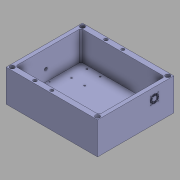
# Autodesk Inventor part: podstawa_2
Saved by Autodesk Inventor 2021 (Build 250183000, 183)
## iProperties
Created: 2022-06-23
Part Number: podstawa_2
Material: PC/ABS Plastic
Document SubType Name: Modeling
Designer: agnpi
Density: 0.357273 g/cm^3
Appearance: Olive Green
Author: agnpi
Autodesk Inventor part; units mm, degrees
ref_plane "YZ Plane" through (0, 0, 0) normal (1, 0, 0) x (0, 1, 0)
ref_plane "XZ Plane" through (0, 0, 0) normal (0, 1, 0) x (-1, 0, 0)
ref_plane "XY Plane" through (0, 0, 0) normal (0, 0, 1) x (1, 0, 0)
sketch "Sketch1" plane through (0, 0, 0) normal (0, 1, 0) x (-1, 0, 0)
  line L0 (179.2, 0) -> (-179.2, 0) projected
  line L1 (0, -144.2) -> (0, 144.2) projected
  line L2 (-120, 95) -> (120, 95)
  line L3 (120, 95) -> (120, -95)
  line L4 (120, -95) -> (-120, -95)
  line L5 (-120, -95) -> (-120, 95)
  line L6 (-120, 95) -> (120, -95) construction
  line L7 (120, 95) -> (-120, -95) construction
  line L8 (-128, 103) -> (128, 103)
  line L9 (128, 103) -> (128, -103)
  line L10 (128, -103) -> (-128, -103)
  line L11 (-128, -103) -> (-128, 103)
  point P0 (0, 0)
  dimension "d0" = 240
  dimension "d1" = 190
  dimension "d2" = 8
  dimension "d3" = 8
  dimension "d4" = 8
  dimension "d5" = 8
  constraints: 20 end point, 3 parallel, 3 perpendicular, 2 horizontal, 2 midpoint
  measures "d0" distance of L3.end L4.end
  measures "d1" distance of L2.end L3.end
  measures "d2" distance between parallel lines of L2 L8
  measures "d3" distance between parallel lines of L10 L4
  measures "d4" distance between parallel lines of L11 L5
  measures "d5" distance between parallel lines of L9 L3
extrude "Extrusion1" add sketch "Sketch1" along normal blind 8 contours L3 L4 L1 L0 | L0 L1 L2 L3 | L1 L4 L5 L0 | L0 L5 L2 L1
extrude "Extrusion2" add sketch "Sketch1" along normal blind 85 contours L9 L10 L1 L4 L3 L0 | L0 L3 L2 L1 L8 L9 | L1 L2 L5 L0 L11 L8 | L10 L11 L0 L5 L4 L1
move faces "Move1" translate (-16, 0, 0) faces at (120, 33.6667, -31.6667)
move faces "Move5" translate (-8, 0, 0) faces at (128, 28.3333, 34.3333)
move faces "Move6" translate (-8, 0, 0) faces at (120, 28.3333, 34.3333)
move faces "Move7" translate (0, 0, -8) faces at (-45.3333, 59.3333, 95)
move faces "Move8" translate (0, 0, -8) faces at (-48, 28.3333, 103)
move faces "Move9" translate (0, 0, -8) faces at (-45.3333, 59.3333, 87)
move faces "Move10" translate (0, 0, -8) faces at (-48, 28.3333, 95)
thicken "Thicken1" operation add thickness 3 both sides no extend neighbours yes toward (0, 0, 1) faces at (-48, 28.3333, 87)
thicken "Thicken3" operation add thickness 3 both sides no extend neighbours yes toward (0, 0, -1) faces at (32, 28.3333, -103)
sketch "Sketch5" plane through (0, 8, 0) normal (0, 1, 0) x (1, 0, 0)
  line L0 (-120, -79) -> (-120, 95) projected
  line L1 (-120, 95) -> (104, 95) projected
  line L2 (-120, 89.3431) -> (-114.3431, 95)
  line L3 (-120, 89.3431) -> (-120, 95)
  line L4 (98.3431, 95) -> (104, 89.3431)
  line L5 (104, 95) -> (104, -79) projected
  line L6 (-120, -73.3431) -> (-114.3431, -79)
  line L7 (104, -79) -> (-120, -79) projected
  line L8 (98.3431, -79) -> (104, -73.3431)
  point P0 (0, 0)
  dimension "d69" = 45
  dimension "d70" = 8
  dimension "d73" = 8
  dimension "d74" = 45
  dimension "d75" = 8
  dimension "d76" = 45
  dimension "d77" = 8
  dimension "d78" = 45
  constraints: 10 end point, 8 point on line, 1 collinear
  measures "d69" angle of L2 L0
  measures "d70" distance of L2.start L2.end
  measures "d73" distance of L4.start L4.end
  measures "d74" angle of L5 L4
  measures "d75" distance of L6.start L6.end
  measures "d76" angle of L7 L6
  measures "d77" distance of L8.start L8.end
  measures "d78" angle of L7 L8
thicken "Thicken4" operation add thickness 1 both sides no extend neighbours yes toward (1, 0, 0) faces at (-120, 59.3333, 21)
thicken "Thicken5" operation add thickness 1 both sides no extend neighbours yes toward (-1, 0, 0) faces at (104, 33.6667, 21)
extrude "Extrusion6" add sketch "Sketch5" along normal up to surface (77 mm away) contours L0 L6 L7 | L0 L1 L2 | L8 L5 L7 | L1 L5 L4
sketch "Sketch7" plane through (0, 8, 0) normal (0, 1, 0) x (1, 0, 0)
  line L0 (-119, -74.3431) -> (-119, 90.3431) projected
  line L1 (-114.3431, 95) -> (98.3431, 95) projected
  point P0 (0, 0)
  point P1 (-94.5, 86.37)
  point P2 (-59.5, 86.37)
  point P3 (-94.5, 45.37)
  point P4 (-59.5, 45.37)
  dimension "d95" = 24.5
  dimension "d96" = 24.5
  dimension "d97" = 41
  dimension "d98" = 35
  dimension "d99" = 35
  dimension "d100" = 8.63
  dimension "d101" = 8.63
  dimension "d102" = 41
  measures "d95" distance from line of L0 point (-94.5, 86.37)
  measures "d96" distance from line of L0 point (-94.5, 45.37)
  measures "d97" distance of point (-94.5, 86.37) point (-94.5, 45.37)
  measures "d98" distance of point (-59.5, 45.37) point (-94.5, 45.37)
  measures "d99" distance of point (-59.5, 86.37) point (-94.5, 86.37)
  measures "d100" distance from line of L1 point (-59.5, 86.37)
  measures "d101" distance from line of L1 point (-94.5, 86.37)
  measures "d102" distance of point (-59.5, 45.37) point (-59.5, 86.37)
hole "Hole2" at (-94.5, 8, -86.37) at (-59.5, 8, -86.37) at (-94.5, 8, -45.37) at (-59.5, 8, -45.37) direction (0, -1, 0) diameter 4 end through all
sketch "Sketch8" plane through (0, 8, 0) normal (0, 1, 0) x (1, 0, 0)
  line L0 (-114.3431, 95) -> (98.3431, 95) projected
  line L1 (103, 90.3431) -> (103, -74.3431) projected
  point P0 (0, 0)
  point P1 (29, 66.38)
  point P2 (71, 66.37)
  point P3 (38.2, 51.57)
  point P4 (66.91, 51.57)
  dimension "d110" = 28.71
  dimension "d111" = 28.63
  dimension "d112" = 28.62
  dimension "d113" = 43.43
  dimension "d114" = 43.43
  dimension "d115" = 74
  dimension "d116" = 42
  dimension "d117" = 64.8
  measures "d110" distance of point (66.91, 51.57) point (38.2, 51.57)
  measures "d111" distance from line of L0 point (71, 66.37)
  measures "d112" distance from line of L0 point (29, 66.38)
  measures "d113" distance from line of L0 point (66.91, 51.57)
  measures "d114" distance from line of L0 point (38.2, 51.57)
  measures "d115" distance from line of L1 point (29, 66.38)
  measures "d116" distance of point (71, 66.37) point (29, 66.38)
  measures "d117" distance from line of L1 point (38.2, 51.57)
hole "Hole3" at (29, 8, -66.38) at (71, 8, -66.37) at (38.2, 8, -51.57) at (66.91, 8, -51.57) direction (0, -1, 0) diameter 4 end through all
sketch "Sketch9" plane through (0, 8, 0) normal (0, 1, 0) x (1, 0, 0)
  line L0 (103, 90.3431) -> (103, -74.3431) projected
  line L1 (98.3431, -79) -> (-114.3431, -79) projected
  point P0 (0, 0)
  point P1 (35, 18.8)
  point P2 (70, 18.8)
  point P3 (35, -14.2)
  point P4 (70, -14.2)
  dimension "d125" = 33
  dimension "d126" = 33
  dimension "d127" = 35
  dimension "d128" = 35
  dimension "d129" = 33
  dimension "d130" = 33
  dimension "d131" = 64.8
  dimension "d132" = 64.8
  measures "d125" distance from line of L0 point (70, 18.8)
  measures "d126" distance from line of L0 point (70, -14.2)
  measures "d127" distance of point (70, 18.8) point (35, 18.8)
  measures "d128" distance of point (70, -14.2) point (35, -14.2)
  measures "d129" distance of point (35, -14.2) point (35, 18.8)
  measures "d130" distance of point (70, -14.2) point (70, 18.8)
  measures "d131" distance from line of L1 point (35, -14.2)
  measures "d132" distance from line of L1 point (70, -14.2)
hole "Hole4" at (35, 8, -18.8) at (70, 8, -18.8) at (35, 8, 14.2) at (70, 8, 14.2) direction (0, -1, 0) diameter 4 end through all
sketch "Sketch10" plane through (0, 8, 0) normal (0, 1, 0) x (1, 0, 0)
  line L0 (-119, -74.3431) -> (-119, 90.3431) projected
  line L1 (98.3431, -79) -> (-114.3431, -79) projected
  point P0 (0, 0)
  point P1 (-115, 7.85)
  point P2 (-115, -4.15)
  dimension "d140" = 4
  dimension "d141" = 4
  dimension "d142" = 74.85
  dimension "d143" = 12
  measures "d140" distance from line of L0 point (-115, -4.15)
  measures "d141" distance from line of L0 point (-115, 7.85)
  measures "d142" distance from line of L1 point (-115, -4.15)
  measures "d143" distance of point (-115, 7.85) point (-115, -4.15)
hole "Hole5" at (-115, 8, -7.85) at (-115, 8, 4.15) direction (0, -1, 0) diameter 3 end through all
move faces "Move21" translate (0, 0, 3) faces at (-48, 28.3333, 90)
move faces "Move22" translate (0, 0, -3) faces at (-48, 56.6667, -106)
move faces "Move23" translate (1, 0, 0) faces at (112, 56.6667, -41.6667)
move faces "Move24" translate (-1, 0, 0) faces at (-128, 28.3333, -41.6667)
sketch "Sketch15" plane through (0, 85, 0) normal (0, 1, 0) x (1, 0, 0)
  circle A0 centre (-121, 101) radius 6
  line L0 (113, 109) -> (-129, 109) projected
  line L1 (-129, 109) -> (-129, -93) projected
  circle A1 centre (105, 101) radius 6
  line L2 (113, -93) -> (113, 109) projected
  circle A2 centre (105, -85) radius 6
  line L3 (-129, -93) -> (113, -93) projected
  circle A3 centre (-121, -85) radius 6
  point P0 (0, 0)
  dimension "d204" = 12
  dimension "d205" = 8
  dimension "d206" = 8
  dimension "d207" = 12
  dimension "d208" = 8
  dimension "d209" = 8
  dimension "d210" = 12
  dimension "d211" = 8
  dimension "d212" = 8
  dimension "d213" = 12
  dimension "d214" = 8
  dimension "d215" = 8
  constraints: 4 centre point
  measures "d204" diameter of A0
  measures "d205" distance from line of L0 A0.centre
  measures "d206" distance from line of L1 A0.centre
  measures "d207" diameter of A1
  measures "d208" distance from line of L2 A1.centre
  measures "d209" distance from line of L0 A1.centre
  measures "d210" diameter of A2
  measures "d211" distance from line of L2 A2.centre
  measures "d212" distance from line of L3 A2.centre
  measures "d213" diameter of A3
  measures "d214" distance from line of L3 A3.centre
  measures "d215" distance from line of L1 A3.centre
extrude "Extrusion7" cut sketch "Sketch15" against normal blind 15 contours A0 | A1 | A2 | A3
sketch "Sketch16" plane through (-129, 0, -109) normal (-1, 0, 0) x (0, 0, 1)
  circle A0 centre (107.1, 38) radius 4
  line L0 (202, 0) -> (202, 85) projected
  line L1 (0, 0) -> (202, 0) projected
  point P0 (109, 0)
  dimension "d218" = 8
  dimension "d219" = 94.9
  dimension "d220" = 38
  constraints: 1 centre point
  measures "d218" diameter of A0
  measures "d219" distance from line of L0 A0.centre
  measures "d220" distance from line of L1 A0.centre
extrude "Extrusion8" cut sketch "Sketch16" against normal up to surface (10 mm away)
sketch "Sketch17" plane through (0, 85, 0) normal (0, 1, 0) x (1, 0, 0)
  circle A0 centre (-60, -86) radius 4.5
  circle A1 centre (105, -85) radius 6 projected
  line L0 (-129, -93) -> (113, -93) projected
  circle A2 centre (-60, 102) radius 4.5
  line L1 (113, 109) -> (-129, 109) projected
  circle A3 centre (105, 101) radius 6 projected
  circle A4 centre (-121, -85) radius 6 projected
  circle A5 centre (-121, 101) radius 6 projected
  point P0 (0, 0)
  dimension "d223" = 9
  dimension "d225" = 7
  dimension "d226" = 9
  dimension "d227" = 7
  dimension "d231" = 61
  dimension "d232" = 61
  constraints: 2 centre point
  measures "d223" diameter of A0
  measures "d225" distance from line of L0 A0.centre
  measures "d226" diameter of A2
  measures "d227" distance from line of L1 A2.centre
  measures "d231" horizontal distance of A4.centre A0.centre
  measures "d232" horizontal distance of A5.centre A2.centre
extrude "Extrusion9" cut sketch "Sketch17" against normal blind 15 contours A0 | A2
sketch "Sketch18" plane through (0, 85, 0) normal (0, 1, 0) x (1, 0, 0)
  circle A0 centre (-15, -86) radius 4
  circle A1 centre (-15, 102) radius 4
  circle A2 centre (105, -85) radius 6 projected
  circle A3 centre (105, 101) radius 6 projected
  line L0 (113, 109) -> (-129, 109) projected
  line L1 (-129, -93) -> (113, -93) projected
  point P0 (0, 0)
  dimension "d233" = 8
  dimension "d234" = 8
  dimension "d235" = 120
  dimension "d236" = 120
  dimension "d237" = 7
  dimension "d238" = 7
  constraints: 2 centre point
  measures "d233" diameter of A0
  measures "d234" diameter of A1
  measures "d235" horizontal distance of A0.centre A2.centre
  measures "d236" horizontal distance of A1.centre A3.centre
  measures "d237" distance from line of L0 A1.centre
  measures "d238" distance from line of L1 A0.centre
extrude "Extrusion10" cut sketch "Sketch18" against normal blind 15 contours A0 | A1
sketch "Sketch19" plane through (-129, 0, -109) normal (-1, 0, 0) x (0, 0, 1)
  line L0 (162, 45) -> (182, 45)
  line L1 (182, 45) -> (182, 25)
  line L2 (182, 25) -> (162, 25)
  line L3 (162, 25) -> (162, 45)
  line L4 (202, 0) -> (202, 85) projected
  line L5 (0, 0) -> (202, 0) projected
  point P0 (109, 0)
  dimension "d241" = 20
  dimension "d242" = 20
  dimension "d243" = 45
  dimension "d244" = 25
  constraints: 8 end point, 2 parallel, 1 horizontal, 1 perpendicular
  measures "d241" distance between parallel lines of L4 L1
  measures "d242" distance between parallel lines of L3 L1
  measures "d243" distance between parallel lines of L5 L0
  measures "d244" distance between parallel lines of L5 L2
extrude "Extrusion11" cut sketch "Sketch19" against normal up to surface (10 mm away)
sketch "Sketch20" plane through (103, 8, -90.3431) normal (-1, 0, 0) x (0, 0, 1)
  line L0 (20, 66) -> (45.5, 66)
  line L1 (45.5, 66) -> (45.5, 63)
  line L2 (45.5, 63) -> (20, 63)
  line L3 (20, 63) -> (20, 66)
  line L4 (20, 63) -> (17, 63)
  line L5 (17, 63) -> (17, 37.5)
  line L6 (17, 37.5) -> (20, 37.5)
  line L7 (20, 37.5) -> (20, 63)
  line L8 (20, 37.5) -> (45.5, 37.5)
  line L9 (45.5, 37.5) -> (45.5, 34.5)
  line L10 (45.5, 34.5) -> (20, 34.5)
  line L11 (20, 34.5) -> (20, 37.5)
  line L12 (45.5, 63) -> (48.5, 63)
  line L13 (48.5, 63) -> (48.5, 37.5)
  line L14 (48.5, 37.5) -> (45.5, 37.5)
  line L15 (45.5, 37.5) -> (45.5, 63)
  line L16 (0, 77) -> (164.6863, 77) projected
  line L17 (0, 77) -> (0, 0) projected
  point P0 (90.3431, -8)
  dimension "d247" = 3
  dimension "d248" = 14
  dimension "d249" = 25.5
  dimension "d250" = 25.5
  dimension "d251" = 25.5
  dimension "d252" = 25.5
  dimension "d253" = 3
  dimension "d254" = 3
  dimension "d255" = 3
  dimension "d256" = 20
  constraints: 32 end point, 8 parallel, 4 horizontal, 4 perpendicular, 1 point on line
  measures "d247" distance between parallel lines of L2 L0
  measures "d248" distance between parallel lines of L16 L2
  measures "d249" distance of L1.end L2.end
  measures "d250" distance of L4.end L5.end
  measures "d251" distance of L9.end L10.end
  measures "d252" distance of L12.end L13.end
  measures "d253" distance between parallel lines of L8 L10
  measures "d254" distance between parallel lines of L7 L5
  measures "d255" distance between parallel lines of L13 L15
  measures "d256" distance from line of L17 L2.end
extrude "Extrusion12" add sketch "Sketch20" along normal blind 3 contours L0 L1 L2 L3 | L7 L6 L5 L4 | L12 L13 L14 L15 | L8 L9 L10 L11
sketch "Sketch21" plane through (103, 45.5, -70.3431) normal (-1, 0, 0) x (0, 0, 1)
  circle A0 centre (2.75, 2.75) radius 1.5
  circle A1 centre (2.75, 22.75) radius 1.5
  circle A2 centre (22.75, 22.75) radius 1.5
  circle A3 centre (22.75, 2.75) radius 1.5
  line L0 (0, 25.5) -> (25.5, 25.5) projected
  line L1 (0, 0) -> (0, 25.5) projected
  line L2 (0, 0) -> (25.5, 0) projected
  line L3 (25.5, 25.5) -> (25.5, 0) projected
  point P0 (70.3431, -45.5)
  dimension "d259" = 3
  dimension "d260" = 3
  dimension "d261" = 3
  dimension "d262" = 3
  dimension "d263" = 2.75
  dimension "d264" = 2.75
  dimension "d265" = 2.75
  dimension "d266" = 2.75
  dimension "d267" = 2.75
  dimension "d268" = 2.75
  dimension "d269" = 2.75
  dimension "d270" = 2.75
  constraints: 4 centre point
  measures "d259" diameter of A0
  measures "d260" diameter of A1
  measures "d261" diameter of A2
  measures "d262" diameter of A3
  measures "d263" distance from line of L0 A1.centre
  measures "d264" distance from line of L1 A1.centre
  measures "d265" distance from line of L2 A0.centre
  measures "d266" distance from line of L1 A0.centre
  measures "d267" distance from line of L0 A2.centre
  measures "d268" distance from line of L3 A3.centre
  measures "d269" distance from line of L2 A3.centre
  measures "d270" distance from line of L3 A2.centre
extrude "Extrusion13" cut sketch "Sketch21" against normal through all contours A0 | A1 | A2 | A3
sketch "Sketch22" plane through (113, 0, 93) normal (1, 0, 0) x (0, 0, -1)
  line L0 (137.8431, 71) -> (137.8431, 74) projected
  line L1 (163.3431, 71) -> (163.3431, 45.5) projected
  line L2 (137.8431, 71) -> (163.3431, 71)
  line L3 (163.3431, 71) -> (163.3431, 45.5)
  line L4 (163.3431, 45.5) -> (137.8431, 45.5)
  line L5 (137.8431, 45.5) -> (137.8431, 71)
  circle A0 centre (150.5931, 58.25) radius 6
  circle A1 centre (150.5931, 58.25) radius 11.5
  line L6 (146.0144, 62.1275) -> (142.0931, 65.996)
  line L7 (147.1208, 63.1431) -> (143.174, 67.0367)
  line L8 (144.9458, 56.2234) -> (139.6349, 54.7618)
  line L9 (144.6194, 57.6894) -> (139.2741, 56.2182)
  line L10 (149.5245, 52.3459) -> (148.1349, 47.0158)
  line L11 (148.0918, 52.7963) -> (146.6932, 47.4315)
  line L12 (155.1719, 54.3725) -> (159.0931, 50.504)
  line L13 (154.0655, 53.3569) -> (158.0123, 49.4633)
  line L14 (156.2405, 60.2766) -> (161.5513, 61.7382)
  line L15 (156.5669, 58.8106) -> (161.9122, 60.2818)
  line L16 (151.6618, 64.1541) -> (153.0513, 69.4842)
  line L17 (153.0945, 63.7037) -> (154.4931, 69.0685)
  circle A2 centre (150.5931, 58.25) radius 6.75
  circle A3 centre (150.5931, 58.25) radius 7.5
  circle A4 centre (150.5931, 58.25) radius 8.25
  circle A5 centre (150.5931, 58.25) radius 9
  circle A6 centre (150.5931, 58.25) radius 9.75
  circle A7 centre (150.5931, 58.25) radius 10.5
  point P0 (93, 0)
  point P1 (157.6901, 60.6755)
  point P2 (153.4776, 65.1731)
  point P3 (153.2863, 64.4395)
  point P4 (156.9655, 60.4761)
  point P5 (156.2422, 53.3166)
  point P6 (158.031, 59.2136)
  point P7 (157.3, 59.0124)
  point P8 (155.7072, 53.8444)
  point P9 (149.1452, 50.8911)
  point P10 (155.1465, 52.2904)
  point P11 (154.6068, 52.8229)
  point P12 (149.3348, 51.6183)
  point P13 (143.4962, 55.8245)
  point P14 (147.7087, 51.3269)
  point P15 (147.9, 52.0605)
  point P16 (144.2208, 56.0239)
  point P17 (144.9441, 63.1834)
  point P18 (143.1553, 57.2864)
  point P19 (143.8863, 57.4876)
  point P20 (145.4791, 62.6556)
  point P21 (152.0411, 65.6089)
  point P22 (146.0397, 64.2096)
  point P23 (146.5795, 63.6771)
  point P24 (151.8515, 64.8817)
  point P25 (142.0477, 55.4258)
  point P26 (147.3272, 49.8635)
  point P27 (147.5178, 50.5946)
  point P28 (142.7719, 55.6251)
  point P29 (148.7663, 49.4374)
  point P30 (156.2231, 51.2284)
  point P31 (155.6852, 51.759)
  point P32 (148.9557, 50.1641)
  point P33 (159.4891, 59.6149)
  point P34 (158.7606, 59.4144)
  point P35 (156.777, 52.789)
  point P36 (157.3117, 52.2615)
  point P37 (159.1386, 61.0742)
  point P38 (153.8591, 66.6365)
  point P39 (153.6685, 65.9054)
  point P40 (158.4144, 60.8749)
  point P41 (152.42, 67.0626)
  point P42 (144.9632, 65.2716)
  point P43 (145.5011, 64.741)
  point P44 (152.2306, 66.3359)
  point P45 (143.8746, 64.2385)
  point P46 (141.6972, 56.8851)
  point P47 (142.4257, 57.0856)
  point P48 (144.4093, 63.711)
  point P49 (152.7989, 68.5157)
  point P50 (143.8891, 66.3312)
  point P51 (144.4259, 65.8017)
  point P52 (152.6095, 67.7892)
  point P53 (160.5864, 61.4726)
  point P54 (154.2397, 68.0965)
  point P55 (154.0495, 67.3668)
  point P56 (159.8625, 61.2734)
  point P57 (160.9437, 60.0152)
  point P58 (160.2167, 59.8151)
  point P59 (157.8462, 51.7342)
  point P60 (158.3807, 51.2069)
  point P61 (148.3874, 47.9843)
  point P62 (157.2971, 50.1688)
  point P63 (156.7604, 50.6983)
  point P64 (148.5768, 48.7108)
  point P65 (142.8056, 65.2931)
  point P66 (140.2426, 56.4848)
  point P67 (140.9696, 56.6849)
  point P68 (143.3401, 64.7658)
  point P69 (140.5999, 55.0274)
  point P70 (146.9466, 48.4035)
  point P71 (147.1368, 49.1332)
  point P72 (141.3238, 55.2266)
  dimension "d273" = 12
  dimension "d274" = 12.75
  dimension "d275" = 12.75
  dimension "d277" = 23
  dimension "d283" = 1.5
  dimension "d284" = 3.9633
  dimension "d285" = 5.004
  dimension "d288" = 360
  dimension "d290" = 13.5
  dimension "d291" = 15
  dimension "d298" = 16.5
  dimension "d299" = 18
  dimension "d300" = 19.5
  dimension "d301" = 21
  constraints: 32 end point, 8 centre point, 6 coincident, 4 point on circle, 3 parallel, 1 concentric, 1 horizontal, 1 perpendicular, 37 other
  measures "d273" diameter of A0
  measures "d274" distance from line of L5 A0.centre
  measures "d275" distance from line of L4 A0.centre
  measures "d277" diameter of A1
  measures "d283" distance between parallel lines of L7 L6
  measures "d284" distance from line of L2 L7.end
  measures "d285" distance from line of L2 L6.end
  measures "d290" diameter of A2
  measures "d291" diameter of A3
  measures "d298" diameter of A4
  measures "d299" diameter of A5
  measures "d300" diameter of A6
  measures "d301" diameter of A7
extrude "Extrusion14" cut sketch "Sketch22" against normal up to surface (10 mm away) contours A0 | A0 L15 A2 L12 | A0 L14 A2 L15 | L12 A2 L13 A0 | A0 L17 A2 L14 | A2 L14 A3 L15 | L15 A3 L12 A2 | L13 A2 L10 A0 | L12 A3 L13 A2 | A0 L16 A2 L17 | A2 L17 A3 L14 | A3 L14 A4 L15 | L15 A4 L12 A3 | L10 A2 L11 A0 | L13 A3 L10 A2 | L12 A4 L13 A3 | A0 L7 A2 L16 | A2 L16 A3 L17 | A3 L17 A4 L14 | A4 L14 A5 L15 | L15 A5 L12 A4 | L11 A2 L8 A0 | L10 A3 L11 A2 | L13 A4 L10 A3 | L12 A5 L13 A4 | A0 L6 A2 L7 | A2 L7 A3 L16 | A3 L16 A4 L17 | A4 L17 A5 L14 | A5 L14 A6 L15 | L15 A6 L12 A5 | L8 A2 L9 A0 | L11 A3 L8 A2 | L10 A4 L11 A3 | L13 A5 L10 A4 | L12 A6 L13 A5 | A0 L9 A2 L6 | A2 L6 A3 L7 | A3 L7 A4 L16 | A4 L16 A5 L17 | A5 L17 A6 L14 | A6 L14 A7 L15 | L15 A7 L12 A6 | L8 A3 L9 A2 | L11 A4 L8 A3 | L10 A5 L11 A4 | L13 A6 L10 A5 | L12 A7 L13 A6 | A2 L9 A3 L6 | A3 L6 A4 L7 | A4 L7 A5 L16 | A5 L16 A6 L17 | A6 L17 A7 L14 | A7 L14 A1 L15 | L15 A1 L12 A7 | L8 A4 L9 A3 | L11 A5 L8 A4 | L10 A6 L11 A5 | L13 A7 L10 A6 | L12 A1 L13 A7 | A3 L9 A4 L6 | A4 L6 A5 L7 | A5 L7 A6 L16 | A6 L16 A7 L17 | A7 L17 A1 L14 | L8 A5 L9 A4 | L11 A6 L8 A5 | L10 A7 L11 A6 | L13 A1 L10 A7 | A4 L9 A5 L6 | A5 L6 A6 L7 | A6 L7 A7 L16 | A7 L16 A1 L17 | L8 A6 L9 A5 | L11 A7 L8 A6 | L10 A1 L11 A7 | A5 L9 A6 L6 | A6 L6 A7 L7 | A7 L7 A1 L16 | L8 A7 L9 A6 | L11 A1 L8 A7 | A6 L9 A7 L6 | A7 L6 A1 L7 | L8 A1 L9 A7 | A7 L9 A1 L6
extrude "Extrusion15" add sketch "Sketch22" against normal blind 1 contours A0
extrude "Extrusion16" add sketch "Sketch22" against normal blind 1 contours A0 L14 A2 L15 | L12 A2 L13 A0 | A2 L14 A3 L15 | L12 A3 L13 A2 | A0 L16 A2 L17 | A3 L14 A4 L15 | L10 A2 L11 A0 | L12 A4 L13 A3 | A2 L16 A3 L17 | A4 L14 A5 L15 | L10 A3 L11 A2 | L12 A5 L13 A4 | A0 L6 A2 L7 | A3 L16 A4 L17 | A5 L14 A6 L15 | L8 A2 L9 A0 | L10 A4 L11 A3 | L12 A6 L13 A5 | A2 L6 A3 L7 | A4 L16 A5 L17 | A6 L14 A7 L15 | L8 A3 L9 A2 | L10 A5 L11 A4 | L12 A7 L13 A6 | A3 L6 A4 L7 | A5 L16 A6 L17 | A7 L14 A1 L15 | L8 A4 L9 A3 | L10 A6 L11 A5 | L12 A1 L13 A7 | A4 L6 A5 L7 | A6 L16 A7 L17 | L8 A5 L9 A4 | L10 A7 L11 A6 | A5 L6 A6 L7 | A7 L16 A1 L17 | L8 A6 L9 A5 | L10 A1 L11 A7 | A6 L6 A7 L7 | L8 A7 L9 A6 | A7 L6 A1 L7 | L8 A1 L9 A7
extrude "Extrusion17" add sketch "Sketch22" against normal blind 1 contours L15 A3 L12 A2 | A2 L17 A3 L14 | L13 A3 L10 A2 | A2 L7 A3 L16 | L11 A3 L8 A2 | A2 L9 A3 L6
extrude "Extrusion18" add sketch "Sketch22" against normal blind 1 contours L15 A5 L12 A4 | A4 L17 A5 L14 | L13 A5 L10 A4 | A4 L7 A5 L16 | L11 A5 L8 A4 | A4 L9 A5 L6
extrude "Extrusion19" add sketch "Sketch22" against normal blind 1 contours L15 A7 L12 A6 | A6 L17 A7 L14 | L13 A7 L10 A6 | A6 L7 A7 L16 | L11 A7 L8 A6 | A6 L9 A7 L6
body "Solid1"
